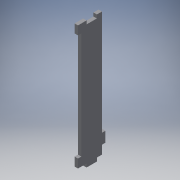
# Autodesk Inventor part: Part2
Saved by Autodesk Inventor 2018 (Build 220112000, 112)
## iProperties
Created: 2018-05-22
Part Number: Part2
Material: Generic
Document SubType Name: Modeling
Designer: Administrator
Density: 1 g/cm^3
Appearance: Default
Author: Administrator
Autodesk Inventor part; units mm, degrees
ref_plane "YZ Plane" through (0, 0, 0) normal (1, 0, 0) x (0, 1, 0)
ref_plane "XZ Plane" through (0, 0, 0) normal (0, 1, 0) x (-1, 0, 0)
ref_plane "XY Plane" through (0, 0, 0) normal (0, 0, 1) x (1, 0, 0)
sketch "Sketch1" plane through (0, 0, 0) normal (1, 0, 0) x (0, 1, 0)
  line L0 (90.5542, 74.5762) -> (-23.7458, 74.5762)
  line L1 (-23.7458, 74.5762) -> (-23.7458, 49.1762)
  line L2 (-23.7458, 49.1762) -> (90.5542, 49.1762)
  line L3 (90.5542, 49.1762) -> (90.5542, 74.5762)
  line L4 (-23.7458, 66.6387) -> (-26.9208, 66.6387)
  line L5 (-26.9208, 66.6387) -> (-26.9208, 57.1137)
  line L6 (-26.9208, 57.1137) -> (-23.7458, 57.1137)
  line L7 (-23.7458, 57.1137) -> (-23.7458, 66.6387)
  point P0 (0, 0)
  dimension "d0" = 25.4
  dimension "d1" = 114.3
  dimension "d4" = 3.175
  dimension "d5" = 7.9375
  dimension "d6" = 7.9375
  constraints: 16 end point, 4 parallel, 2 horizontal, 2 perpendicular, 1 point on line
  measures "d0" distance between parallel lines of L2 L0
  measures "d1" distance between parallel lines of L3 L1
  measures "d4" distance between parallel lines of L1 L5
  measures "d5" distance between parallel lines of L2 L6
  measures "d6" distance between parallel lines of L0 L4
extrude "Extrusion2" add sketch "Sketch1" along normal blind 3.175
sketch "Sketch4" plane through (3.175, 0, 0) normal (1, 0, 0) x (0, 0, -1)
  point P0 (0, 0)
body "Solid2"
